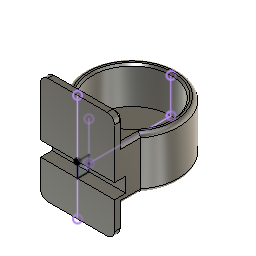
7-pin trailer hitch connector dock (Autodesk Fusion 360 design; units mm, degrees)
Autodesk Fusion 360 part; units mm, degrees
sketch "Sketch1" plane through (0, 0, 0) normal (0, 0, 1) x (1, 0, 0)
  line L0 (0, -21.25) -> (0, 0) construction
  line L1 (-4.5, -20.7681) -> (-4.5, -23.25)
  line L2 (4.5, -20.7681) -> (4.5, -23.25)
  line L3 (4.5, -23.25) -> (-4.5, -23.25)
  arc A0 (4.5, -20.7681) -> (-4.5, -20.7681) centre (0, 0) ccw
  arc A1 (0, -21.25) -> (4.5, -20.7681) centre (0, 0) ccw construction
  arc A2 (-4.5, -20.7681) -> (0, -21.25) centre (0, 0) ccw construction
  arc A3 (5.3471, -24.6773) -> (-5.3471, -24.6773) centre (0, 0) ccw
  line L4 (-20, -15.4131) -> (-20, -29.4131)
  line L5 (20, -15.4131) -> (20, -29.4131)
  line L6 (0, 0) -> (0, 21.25) construction
  line L7 (-20, -29.4131) -> (-17.733, -29.4131)
  line L8 (-17.733, -29.4131) -> (20, -29.4131)
  line L9 (-20, -15.4131) -> (-39.4662, 9.8463)
  line L10 (-39.4662, 9.8463) -> (-39.4662, -7.2104)
  dimension "d1" = 42.5
  dimension "d2" = 9
  dimension "d4" = 4
  dimension "d5" = 44.5
  dimension "d8" = 40
  dimension "d9" = 142.38
  dimension "d10" = 37.62
  dimension "d11" = 14
  constraint coincident L0.end A0.centre
  constraint vertical L0
  constraint parallel L0 L1
  constraint symmetric L0 L1.start L2.start
  constraint symmetric L0 L1.end L2.end
  constraint concentric A0 A1
  constraint concentric A0 A2
  constraint coincident A3 L4.start
  constraint vertical L4
  constraint symmetric L0 L4.start L5.start
  constraint symmetric L0 L4.end L5.end
  constraint midpoint A0 L6.end
  constraint perpendicular L4 L7
  constraint tangent A3 L9
  constraint vertical L10
  measures "d1" diameter of A0
  measures "d2" distance of L1.end L2.end
  measures "d5" distance of L3 L6.end
  measures "d8" distance of L4 L5
  measures "d9" angle of L4 L9 L1.end
  measures "d10" angle of L9 L10 L1.end
  measures "d11" distance of L4.start L4.end L1.end
  measures "d16" distance of L1.end
extrude "Extrude1" add sketch "Sketch1" along normal blind 20 makes body 1
extrude "Extrude2" add sketch "Sketch1" against normal blind 8 contours L1 L2 L3 A0 | A3 L4 L5 L7 L8 bodies 1
sketch "Sketch2" plane through (0, 0, -8) normal (0, 0, -1) x (1, 0, 0)
  arc A0 (-20, 15.4131) -> (20, 15.4131) centre (0, 0) ccw
  line L0 (20, 15.4131) -> (20, 29.4131)
  line L1 (20, 29.4131) -> (-20, 29.4131)
  line L2 (-20, 29.4131) -> (-20, 15.4131)
  line L3 (-20, 15.4131) -> (-20, 29.4131)
  line L4 (20, 15.4131) -> (20, 29.4131)
  line L5 (-17.733, 29.4131) -> (20, 29.4131)
  line L6 (-20, 24.4131) -> (20, 24.4131)
  dimension "d16" = 5
  constraint coincident L2 L6.start
  constraint coincident L0 L6.end
  constraint perpendicular L0 L6
  measures "d16" distance of L1.end L6.start
extrude "Extrude3" add sketch "Sketch2" along normal blind 15 separate body contours L0 L1 L2 L3 L4 L5 L6 makes body 2
fillet "Fillet1" radius 4 2 edges at (20, -26.9131, -23) (-20, -26.9131, -23) on bodies 2
ref_plane "WorkPlane1" through (0, 2.4282, 6) normal (0, 0, 1) x (1, 0, 0)
mirror "Mirror1" about plane through (0, 2.4282, 6) normal (0, 0, 1) of bodies 2 makes body 3
combine "Combine1" operation add target body 1 tool bodies 3 2
fillet "Fillet2" radius 2 6 edges at (20, -19.9131, -8) (0, 25.25, -8) (-20, -19.9131, -8) (0, 25.25, 20) (-20, -19.9131, 20) (20, -19.9131, 20) on bodies 1
chamfer "Chamfer1" distance 1 angle 45 1 edges at (0, 21.25, 20) on bodies 1
chamfer "Chamfer2" distance 2 angle 45 16 edges at (0, -24.4131, 20) (19.4142, -24.4131, 19.4142) (-19.4142, -24.4131, 19.4142) (0, -24.4131, 35) (18.8284, -24.4131, 33.8284) (20, -24.4131, 24.5) (-20, -24.4131, 24.5) (-18.8284, -24.4131, 33.8284) (0, -24.4131, -8) (-19.4142, -24.4131, -7.4142) (19.4142, -24.4131, -7.4142) (0, -24.4131, -23) (18.8284, -24.4131, -21.8284) (20, -24.4131, -12.5) (-20, -24.4131, -12.5) (-18.8284, -24.4131, -21.8284) on bodies 1
sketch "Sketch3" plane through (0, 0, 0) normal (1, 0, 0) x (0, 1, 0)
  line L0 (21.25, 19) -> (21.25, 0)
  line L1 (-23.25, 0) -> (-23.25, 20.8369)
  line L2 (21.25, 0) -> (-23.25, 0)
  line L3 (-29.4131, 35) -> (-29.4131, -23)
  line L4 (-29.4131, 4) -> (-23.25, 4)
  line L5 (-23.25, 4) -> (-23.25, -4)
  line L6 (-23.25, -4) -> (-29.4131, -4)
  line L7 (-29.4131, -4) -> (-29.4131, 4)
  dimension "d27" = 8
  constraint horizontal L4
  constraint vertical L5
  constraint horizontal L6
  constraint vertical L7
  constraint coincident L3 L4.start
  constraint midpoint L1.start L5
  measures "d27" distance of L4.start L6.end
copy_body "Body->Comp1" bodies 1 removing the originals makes body 4 in component "Bottom Draining"
extrude "Extrude1'" cut sketch "Sketch3" along normal through all and the other way through all bodies 4 in component "Bottom Draining"
component "Bottom Draining" placed x (1, 0, 0) y (0, 1, 0) z (0, 0, 1) at (0, 0, 0)
